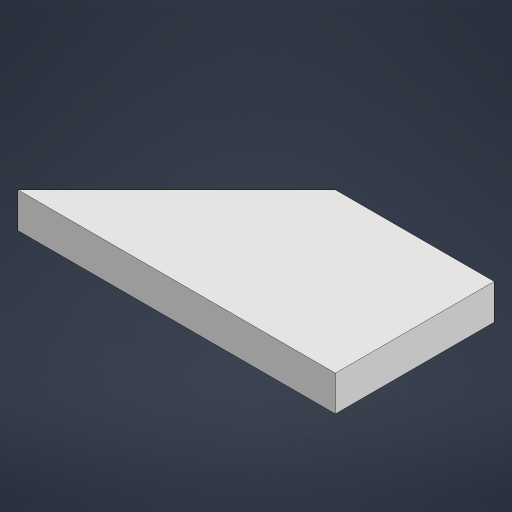
# Autodesk Inventor part: TreadL
Saved by Autodesk Inventor 2023.2 (Build 272271000, 271)
## iProperties
Created: 2022-11-23
Part Number: TreadL
Material: Generic
Document SubType Name: Modeling
Designer: awelt
Mass: 31856.5 g
Surface Area: 8785.94 cm^2
Volume: 31856.5 cm^3
Density: 1 g/cm^3
Appearance: Default
RuleStatus: InUse
BeforeDocSave0: file://C:\Users\awelt\Documents\Inventor\iLogic_Rules\BoundingStore
DocClose0: file://C:\Users\awelt\Documents\Inventor\iLogic_Rules\BoundingStore
Author: awelt
BoundingBL1: 4
BoundingBL2: 18
BoundingBL3: 36
BoundingCF: 1.5
Autodesk Inventor part; units mm, degrees
ref_plane "YZ Plane" through (0, 0, 0) normal (1, 0, 0) x (0, 1, 0)
ref_plane "XZ Plane" through (0, 0, 0) normal (0, 1, 0) x (-1, 0, 0)
ref_plane "XY Plane" through (0, 0, 0) normal (0, 0, 1) x (1, 0, 0)
sketch "Sketch2" plane through (0, 0, 0) normal (0, 1, 0) x (-1, 0, 0)
  line L0 (0, 0) -> (-914.4, 0)
  line L1 (-914.4, 0) -> (-914.4, -457.2)
  line L2 (-914.4, -457.2) -> (0, -457.2)
  line L3 (0, -457.2) -> (0, 0)
  line L4 (0, 0) -> (-457.2, -457.2)
  line L5 (0, 0) -> (646.5784, 0) construction
  dimension "d3" = 914.4
  dimension "d4" = 457.2
  dimension "d5" = 135
  constraints: 12 end point, 2 horizontal, 2 parallel, 1 equal length, 1 midpoint, 1 perpendicular
  measures "d3" distance of L2.end L1.end
  measures "d4" distance of L1.end L0.end
  measures "d5" angle of L4 L5
extrude "Extrusion1" add sketch "Sketch2" along normal blind 101.6 contours L4 L2 L1 L0
body "Solid1"
